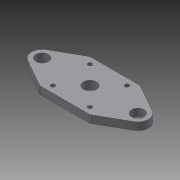
# Autodesk Inventor part: Vertical_Lead_Screw_Shaft_Mount_Plate_Mid
Saved by Autodesk Inventor 2015 (Build 190159000, 159)
## iProperties
Created: 2014-12-22
Part Number: Vertical_Lead_Screw_Shaft_Mount_Plate_Mid
Material: Generic
Document SubType Name: Modeling
Designer: Drew
Density: 1 g/cm^3
Appearance: Default
Author: Drew
Autodesk Inventor part; units mm, degrees
ref_plane "YZ Plane" through (0, 0, 0) normal (1, 0, 0) x (0, 1, 0)
ref_plane "XZ Plane" through (0, 0, 0) normal (0, 1, 0) x (-1, 0, 0)
ref_plane "XY Plane" through (0, 0, 0) normal (0, 0, 1) x (1, 0, 0)
sketch "Sketch1" plane through (0, 0, 0) normal (0, 1, 0) x (-1, 0, 0)
  line L0 (-21, -21) -> (21, -21)
  line L1 (21, -21) -> (21, 21)
  line L2 (21, 21) -> (-21, 21)
  line L3 (-21, 21) -> (-21, -21)
  line L4 (-21, -21) -> (21, 21) construction
  line L5 (21, -21) -> (-21, 21) construction
  circle A0 centre (15.5, 15.5) radius 1.75
  circle A1 centre (0, 0) radius 5.5
  line L6 (34.796, 0) -> (-29.6686, 0)
  line L7 (0, -38.1967) -> (0, 38.2612)
  circle A2 centre (15.5, -15.5) radius 1.75
  circle A3 centre (-15.5, 15.5) radius 1.75
  circle A4 centre (-15.5, -15.5) radius 1.75
  dimension "d0" = 42
  dimension "d1" = 42
  dimension "d4" = 3.5
  dimension "d8" = 11
  dimension "d13" = 31
  constraints: 16 end point, 5 centre point, 3 symmetric about line, 2 horizontal, 2 midpoint, 2 parallel, 1 coincident, 1 perpendicular, 1 point on line, 1 vertical, 3 other
  measures "d0" distance of L0.end L1.end
  measures "d1" distance of L1.end L2.end
  measures "d4" diameter of A0
  measures "d8" diameter of A1
  measures "d13" distance of A2.centre A0.centre
extrude "Extrusion4" add sketch "Sketch1" along normal blind 6.35 contours L3 L6 A1 L7 L0 | L7 A1 L6 L1 L0 | L3 L2 L7 A1 L6 | L6 A1 L7 L2 L1
sketch "Sketch2" plane through (0, 0, 0) normal (0, -1, 0) x (1, 0, 0)
  line L0 (0, 45.4999) -> (0, -47.5937)
  line L1 (43.084, 0) -> (-45.3389, 0)
  arc A0 (-44.3867, 7.7323) -> (-44.3867, -7.7323) centre (-40, 0) ccw
  line L2 (-21, -21) -> (-21, 21) projected
  arc A1 (44.3867, -7.7323) -> (44.3867, 7.7323) centre (40, 0) ccw
  line L3 (-21, 21) -> (-21, -21)
  line L4 (-21, -21) -> (-21, 21) projected
  line L5 (21, 21) -> (21, -21)
  line L6 (21, 21) -> (21, -21) projected
  circle A2 centre (-40, 0) radius 5.25
  circle A3 centre (40, 0) radius 5.25
  line L7 (-21, -21) -> (-44.3867, -7.7323)
  line L8 (-44.3867, 7.7323) -> (-21, 21)
  line L9 (-21, 21) -> (-21, -21)
  line L10 (21, -21) -> (44.3867, -7.7323)
  line L11 (44.3867, 7.7323) -> (21, 21)
  point P0 (0, 0)
  dimension "d18" = 10.5
  dimension "d20" = 80
  dimension "d21" = 8.89
  constraints: 18 end point, 7 symmetric about line, 5 point on circle, 4 centre point, 3 collinear, 2 point on line, 2 tangent, 1 horizontal, 1 vertical, 2 other
  measures "d18" diameter of A2
  measures "d20" distance of A1.centre A2.centre
  measures "d21" radius of A0
extrude "Extrusion5" add sketch "Sketch2" against normal up to surface (6.35 mm away)
fillet "Fillet1" radius 3.175 4 edges at (-21, 3.175, -21) (21, 3.175, -21) (21, 3.175, 21) (-21, 3.175, 21)
equation "\"d0\" = d1"
body "Solid4"
